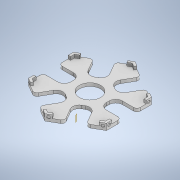
# Autodesk Inventor part: hexlight-bottom-led-module
Saved by Autodesk Inventor 2020 (Build 240168000, 168)
## iProperties
Created: 2019-10-02
Part Number: hexlight-bottom-led-module
Material: Generic
Document SubType Name: Modeling
Designer: Adam
Density: 1 g/cm^3
Appearance: Default
Author: Adam
Autodesk Inventor part; units mm, degrees
ref_plane "YZ Plane" through (0, 0, 0) normal (1, 0, 0) x (0, 1, 0)
ref_plane "XZ Plane" through (0, 0, 0) normal (0, 1, 0) x (-1, 0, 0)
ref_plane "XY Plane" through (0, 0, 0) normal (0, 0, 1) x (1, 0, 0)
sketch "Sketch1" plane through (0, 0, 0) normal (0, 1, 0) x (-1, 0, 0)
  line L0 (73.6122, 42.5) -> (73.6122, -42.5)
  line L1 (73.6122, -42.5) -> (0, -85)
  line L2 (0, -85) -> (-73.6122, -42.5)
  line L3 (-73.6122, -42.5) -> (-73.6122, 42.5)
  line L4 (-73.6122, 42.5) -> (0, 85)
  line L5 (0, 85) -> (73.6122, 42.5)
  point P0 (0, 0)
  point P1 (0, 0)
  dimension "d1" = 0
  dimension "d2" = 85
  constraints: 12 end point, 1 coincident, 13 other
  measures "d1" horizontal distance of point (0, 0) L4.end
  measures "d2" distance of L0.start L0.end
extrude "Extrusion1" add sketch "Sketch1" along normal blind 12
sketch "Sketch2" plane through (0, 12, 0) normal (0, 1, 0) x (1, 0, 0)
  line L0 (-69.282, -40) -> (-69.282, 40)
  line L1 (-69.282, 40) -> (0, 80)
  line L2 (0, 80) -> (69.282, 40)
  line L3 (69.282, 40) -> (69.282, -40)
  line L4 (69.282, -40) -> (0, -80)
  line L5 (0, -80) -> (-69.282, -40)
  point P0 (0, 0)
  point P1 (0, 0)
  dimension "d5" = 0
  dimension "d6" = 80
  constraints: 12 end point, 1 coincident, 13 other
  measures "d5" horizontal distance of point (0, 0) L4.end
  measures "d6" distance of L0.start L0.end
extrude "Extrusion2" cut sketch "Sketch2" against normal blind 6
sketch "Sketch6" plane through (73.6122, 0, 42.5) normal (0.5, 0, 0.8660254) x (0.8660254, 0, -0.5)
  line L0 (-75, 12) -> (-10, 12)
  line L1 (-10, 12) -> (-10, 6)
  line L2 (-10, 6) -> (-75, 6)
  line L3 (-75, 6) -> (-75, 12)
  line L4 (-85, 0) -> (0, 0) projected
  line L5 (-85, 12) -> (0, 12) projected
  line L6 (0, 0) -> (0, 12) projected
  line L7 (-85, 0) -> (-85, 12) projected
  line L8 (-82.5, 6) -> (-2.5, 6) projected
  point P0 (-42.5, 0)
  dimension "d34" = 0
  dimension "d35" = 10
  dimension "d36" = 10
  dimension "d37" = 0
  constraints: 8 end point, 2 parallel, 1 horizontal, 1 perpendicular
  measures "d34" distance between parallel lines of L5 L0
  measures "d35" distance between parallel lines of L6 L1
  measures "d36" distance between parallel lines of L7 L3
  measures "d37" distance between parallel lines of L8 L2
extrude "Extrusion4" cut sketch "Sketch6" against normal blind 11 contours L0 L1 L2 L3
pattern_circular "Circular Pattern2" count 6 over 360 about axis through (0, -10, 0) along (0, 1, 0) of "Extrusion4"
sketch "Sketch7" plane through (0, 0, 85) normal (0.5, 0, 0.8660254) x (0.8660254, 0, -0.5)
  line L0 (0, 0) -> (0, 12) projected
  line L1 (0, 12) -> (10, 12) projected
  point P0 (42.5, 0)
  point P1 (5, 7)
  dimension "d43" = 5
  dimension "d44" = 5
  measures "d43" distance from line of L0 point (5, 7)
  measures "d44" distance from line of L1 point (5, 7)
hole "Hole2" at (4.3301, 7, 82.5) direction (-0.5, 0, -0.8660254) diameter 5.5 depth 1.5
ref_plane "Work Plane1" through (36.8061, 6, 63.75) normal (0.8660254, 0, -0.5) x (-0.5, 0, -0.8660254)
mirror "Mirror1" about plane through (36.8061, 6, 63.75) normal (0.8660254, 0, -0.5) of "Hole2"
pattern_circular "Circular Pattern3" count 6 over 360 about axis through (0, -10, 0) along (0, 1, 0) of "Hole2", "Mirror1"
sketch "Sketch9" plane through (0, 0, 0) normal (0, -1, 0) x (1, 0, 0)
  line L0 (73.6122, 15) -> (46.1122, 15)
  line L1 (33.6122, 2.5) -> (33.6122, -2.5)
  line L2 (46.1122, -15) -> (73.6122, -15)
  line L3 (73.6122, -15) -> (73.6122, 15)
  line L4 (73.6122, 42.5) -> (73.6122, -42.5) projected
  arc A0 (33.6122, -2.5) -> (46.1122, -15) centre (46.1122, -2.5) ccw
  arc A1 (46.1122, 15) -> (33.6122, 2.5) centre (46.1122, 2.5) ccw
  point P0 (0, 0)
  dimension "d64" = 0
  dimension "d65" = 15
  dimension "d67" = 15
  dimension "d68" = 40
  dimension "d71" = 25
  dimension "d72" = 25
  constraints: 8 end point, 4 point on circle, 4 tangent, 2 centre point, 2 parallel, 1 horizontal, 1 perpendicular
  measures "d64" distance between parallel lines of L4 L3
  measures "d65" distance from line of point (0, 0) L0
  measures "d67" distance from line of point (0, 0) L2
  measures "d68" distance between parallel lines of L1 L3
  measures "d71" diameter of A0
  measures "d72" diameter of A1
extrude "Extrusion6" cut sketch "Sketch9" against normal blind 6
sketch "Sketch10" plane through (0, 0, 0) normal (0, -1, 0) x (1, 0, 0)
  line L0 (-17.6122, 27) -> (17.3878, 27) construction
  line L1 (17.3878, 27) -> (17.3878, 20.1168) construction
  line L2 (17.3878, 20.1168) -> (-17.6122, 20.1168) construction
  line L3 (-17.6122, 20.1168) -> (-17.6122, 27) construction
  line L4 (-73.6122, -42.5) -> (-73.6122, 42.5) projected
  line L5 (-73.6122, 42.5) -> (0, 85) projected
  line L6 (0, -85) -> (-73.6122, -42.5) projected
  line L7 (-15.0903, 23.8977) -> (-15.4954, 23.8977)
  line L8 (-15.4954, 23.8977) -> (-15.4954, 25.3895)
  line L9 (-15.4954, 25.3895) -> (-16.8983, 25.3895)
  line L10 (-16.8983, 25.3895) -> (-16.8983, 23.8977)
  line L11 (-16.8983, 23.8977) -> (-17.3034, 23.8977)
  line L12 (-17.3034, 23.8977) -> (-17.3034, 26.9457)
  line L13 (-17.3034, 26.9457) -> (-16.8983, 26.9457)
  line L14 (-16.8983, 26.9457) -> (-16.8983, 25.7502)
  line L15 (-16.8983, 25.7502) -> (-15.4954, 25.7502)
  line L16 (-15.4954, 25.7502) -> (-15.4954, 26.9457)
  line L17 (-15.4954, 26.9457) -> (-15.0903, 26.9457)
  line L18 (-15.0903, 26.9457) -> (-15.0903, 23.8977)
  line L19 (-14.4728, 23.8977) -> (-14.4728, 26.9457)
  line L20 (-14.4728, 26.9457) -> (-12.5659, 26.9457)
  line L21 (-12.5659, 26.9457) -> (-12.5659, 26.585)
  line L22 (-12.5659, 26.585) -> (-14.0677, 26.585)
  line L23 (-14.0677, 26.585) -> (-14.0677, 25.7502)
  line L24 (-14.0677, 25.7502) -> (-12.6672, 25.7502)
  line L25 (-12.6672, 25.7502) -> (-12.6672, 25.3895)
  line L26 (-12.6672, 25.3895) -> (-14.0677, 25.3895)
  line L27 (-14.0677, 25.3895) -> (-14.0677, 24.2583)
  line L28 (-14.0677, 24.2583) -> (-12.5659, 24.2583)
  line L29 (-12.5659, 24.2583) -> (-12.5659, 23.8977)
  line L30 (-12.5659, 23.8977) -> (-14.4728, 23.8977)
  line L31 (-10.0144, 23.8977) -> (-10.4788, 23.8977)
  line L32 (-10.4788, 23.8977) -> (-11.2198, 25.1129)
  line L33 (-11.2198, 25.1129) -> (-11.9756, 23.8977)
  line L34 (-11.9756, 23.8977) -> (-12.4128, 23.8977)
  line L35 (-12.4128, 23.8977) -> (-11.4421, 25.4241)
  line L36 (-11.4421, 25.4241) -> (-12.3831, 26.9457)
  line L37 (-12.3831, 26.9457) -> (-11.9188, 26.9457)
  line L38 (-11.9188, 26.9457) -> (-11.1926, 25.7526)
  line L39 (-11.1926, 25.7526) -> (-10.4516, 26.9457)
  line L40 (-10.4516, 26.9457) -> (-10.0144, 26.9457)
  line L41 (-10.0144, 26.9457) -> (-10.9678, 25.4439)
  line L42 (-10.9678, 25.4439) -> (-10.0144, 23.8977)
  line L43 (-7.9223, 23.8977) -> (-9.6883, 23.8977)
  line L44 (-9.6883, 23.8977) -> (-9.6883, 26.9457)
  line L45 (-9.6883, 26.9457) -> (-9.2833, 26.9457)
  line L46 (-9.2833, 26.9457) -> (-9.2833, 24.2583)
  line L47 (-9.2833, 24.2583) -> (-7.9223, 24.2583)
  line L48 (-7.9223, 24.2583) -> (-7.9223, 23.8977)
  line L49 (-6.5415, 23.8977) -> (-7.7222, 23.8977)
  line L50 (-7.7222, 23.8977) -> (-7.7222, 24.2089)
  line L51 (-7.7222, 24.2089) -> (-7.3344, 24.2089)
  line L52 (-7.3344, 24.2089) -> (-7.3344, 26.6344)
  line L53 (-7.3344, 26.6344) -> (-7.7222, 26.6344)
  line L54 (-7.7222, 26.6344) -> (-7.7222, 26.9457)
  line L55 (-7.7222, 26.9457) -> (-6.5415, 26.9457)
  line L56 (-6.5415, 26.9457) -> (-6.5415, 26.6344)
  line L57 (-6.5415, 26.6344) -> (-6.9293, 26.6344)
  line L58 (-6.9293, 26.6344) -> (-6.9293, 24.2089)
  line L59 (-6.9293, 24.2089) -> (-6.5415, 24.2089)
  line L60 (-6.5415, 24.2089) -> (-6.5415, 23.8977)
  spline S0 degree 2 poles (-4.7631, 23.8384) (-5.0867, 23.8384) (-5.6227, 24.036) (-5.8154, 24.2361) knots 0 0 0 1 2 2 2
  spline S1 degree 2 poles (-5.8154, 24.2361) (-6.008, 24.4386) (-6.213, 25.0363) (-6.213, 25.4241) knots 0 0 0 1 2 2 2
  spline S2 degree 2 poles (-6.213, 25.4241) (-6.213, 25.7922) (-6.0056, 26.3751) (-5.8129, 26.5826) knots 0 0 0 1 2 2 2
  spline S3 degree 2 poles (-5.8129, 26.5826) (-5.6276, 26.7826) (-5.0842, 27) (-4.7607, 27) knots 0 0 0 1 2 2 2
  spline S4 degree 2 poles (-4.7607, 27) (-4.6051, 27) (-4.3235, 26.9555) (-4.195, 26.916) knots 0 0 0 1 2 2 2
  spline S5 degree 2 poles (-4.195, 26.916) (-4.0913, 26.8864) (-3.8393, 26.7777) (-3.7628, 26.7382) knots 0 0 0 1 2 2 2
  line L61 (-3.7628, 26.7382) -> (-3.7628, 26.2491)
  line L62 (-3.7628, 26.2491) -> (-3.7974, 26.2491)
  spline S6 degree 2 poles (-3.7974, 26.2491) (-3.8739, 26.3158) (-4.0345, 26.4368) (-4.1827, 26.506) knots 0 0 0 1 2 2 2
  spline S7 degree 2 poles (-4.1827, 26.506) (-4.3062, 26.5677) (-4.6248, 26.6493) (-4.8076, 26.6493) knots 0 0 0 1 2 2 2
  spline S8 degree 2 poles (-4.8076, 26.6493) (-5.2473, 26.6493) (-5.7907, 25.9873) (-5.7907, 25.4365) knots 0 0 0 1 2 2 2
  spline S9 degree 2 poles (-5.7907, 25.4365) (-5.7907, 25.1302) (-5.6474, 24.6708) (-5.5115, 24.5127) knots 0 0 0 1 2 2 2
  spline S10 degree 2 poles (-5.5115, 24.5127) (-5.3806, 24.3546) (-5.0101, 24.1891) (-4.778, 24.1891) knots 0 0 0 1 2 2 2
  spline S11 degree 2 poles (-4.778, 24.1891) (-4.6075, 24.1891) (-4.2667, 24.2385) (-4.1506, 24.2879) knots 0 0 0 1 2 2 2
  line L63 (-4.1506, 24.2879) -> (-4.1506, 25.0759)
  line L64 (-4.1506, 25.0759) -> (-4.857, 25.0759)
  line L65 (-4.857, 25.0759) -> (-4.857, 25.4315)
  line L66 (-4.857, 25.4315) -> (-3.7504, 25.4315)
  line L67 (-3.7504, 25.4315) -> (-3.7504, 24.1002)
  spline S12 degree 2 poles (-3.7504, 24.1002) (-3.827, 24.0656) (-4.0888, 23.9594) (-4.2, 23.9273) knots 0 0 0 1 2 2 2
  spline S13 degree 2 poles (-4.2, 23.9273) (-4.3506, 23.8828) (-4.5927, 23.8384) (-4.7631, 23.8384) knots 0 0 0 1 2 2 2
  line L68 (-1.0285, 23.8977) -> (-1.4336, 23.8977)
  line L69 (-1.4336, 23.8977) -> (-1.4336, 25.3895)
  line L70 (-1.4336, 25.3895) -> (-2.8365, 25.3895)
  line L71 (-2.8365, 25.3895) -> (-2.8365, 23.8977)
  line L72 (-2.8365, 23.8977) -> (-3.2416, 23.8977)
  line L73 (-3.2416, 23.8977) -> (-3.2416, 26.9457)
  line L74 (-3.2416, 26.9457) -> (-2.8365, 26.9457)
  line L75 (-2.8365, 26.9457) -> (-2.8365, 25.7502)
  line L76 (-2.8365, 25.7502) -> (-1.4336, 25.7502)
  line L77 (-1.4336, 25.7502) -> (-1.4336, 26.9457)
  line L78 (-1.4336, 26.9457) -> (-1.0285, 26.9457)
  line L79 (-1.0285, 26.9457) -> (-1.0285, 23.8977)
  line L80 (0.3004, 23.8977) -> (0.3004, 26.585)
  line L81 (0.3004, 26.585) -> (-0.7222, 26.585)
  line L82 (-0.7222, 26.585) -> (-0.7222, 26.9457)
  line L83 (-0.7222, 26.9457) -> (1.7281, 26.9457)
  line L84 (1.7281, 26.9457) -> (1.7281, 26.585)
  line L85 (1.7281, 26.585) -> (0.7055, 26.585)
  line L86 (0.7055, 26.585) -> (0.7055, 23.8977)
  line L87 (0.7055, 23.8977) -> (0.3004, 23.8977)
  line L88 (5.9592, 23.8977) -> (5.5541, 23.8977)
  line L89 (5.5541, 23.8977) -> (5.5541, 26.5233)
  line L90 (5.5541, 26.5233) -> (4.7588, 24.7375)
  line L91 (4.7588, 24.7375) -> (4.5118, 24.7375)
  line L92 (4.5118, 24.7375) -> (3.7238, 26.5233)
  line L93 (3.7238, 26.5233) -> (3.7238, 23.8977)
  line L94 (3.7238, 23.8977) -> (3.3459, 23.8977)
  line L95 (3.3459, 23.8977) -> (3.3459, 26.9457)
  line L96 (3.3459, 26.9457) -> (3.8992, 26.9457)
  line L97 (3.8992, 26.9457) -> (4.66, 25.2488)
  line L98 (4.66, 25.2488) -> (5.396, 26.9457)
  line L99 (5.396, 26.9457) -> (5.9592, 26.9457)
  line L100 (5.9592, 26.9457) -> (5.9592, 23.8977)
  line L101 (6.2482, 23.8977) -> (7.2757, 26.9457)
  line L102 (7.2757, 26.9457) -> (7.7747, 26.9457)
  line L103 (7.7747, 26.9457) -> (8.8022, 23.8977)
  line L104 (8.8022, 23.8977) -> (8.3749, 23.8977)
  line L105 (8.3749, 23.8977) -> (8.0982, 24.7498)
  line L106 (8.0982, 24.7498) -> (6.9349, 24.7498)
  line L107 (6.9349, 24.7498) -> (6.6582, 23.8977)
  line L108 (6.6582, 23.8977) -> (6.2482, 23.8977)
  line L109 (7.9871, 25.0956) -> (7.5153, 26.5307)
  line L110 (7.5153, 26.5307) -> (7.046, 25.0956)
  line L111 (7.046, 25.0956) -> (7.9871, 25.0956)
  line L112 (11.4501, 23.8977) -> (10.9239, 23.8977)
  line L113 (10.9239, 23.8977) -> (9.9606, 25.1104)
  line L114 (9.9606, 25.1104) -> (9.4963, 25.1104)
  line L115 (9.4963, 25.1104) -> (9.4963, 23.8977)
  line L116 (9.4963, 23.8977) -> (9.0912, 23.8977)
  line L117 (9.0912, 23.8977) -> (9.0912, 26.9457)
  line L118 (9.0912, 26.9457) -> (9.8767, 26.9457)
  spline S14 degree 2 poles (9.8767, 26.9457) (10.1385, 26.9457) (10.4917, 26.8888) (10.6522, 26.7851) knots 0 0 0 1 2 2 2
  spline S15 degree 2 poles (10.6522, 26.7851) (10.8128, 26.6814) (10.998, 26.3578) (10.998, 26.1182) knots 0 0 0 1 2 2 2
  spline S16 degree 2 poles (10.998, 26.1182) (10.998, 25.7848) (10.6572, 25.3327) (10.3657, 25.2241) knots 0 0 0 1 2 2 2
  line L119 (10.3657, 25.2241) -> (11.4501, 23.8977)
  spline S17 degree 2 poles (10.5757, 26.0861) (10.5757, 26.2195) (10.4818, 26.4245) (10.383, 26.4912) knots 0 0 0 1 2 2 2
  spline S18 degree 2 poles (10.383, 26.4912) (10.2966, 26.548) (10.0668, 26.5949) (9.8989, 26.5949) knots 0 0 0 1 2 2 2
  line L120 (9.8989, 26.5949) -> (9.4963, 26.5949)
  line L121 (9.4963, 26.5949) -> (9.4963, 25.4488)
  line L122 (9.4963, 25.4488) -> (9.852, 25.4488)
  spline S19 degree 2 poles (9.852, 25.4488) (10.0273, 25.4488) (10.3064, 25.5106) (10.4028, 25.6069) knots 0 0 0 1 2 2 2
  spline S20 degree 2 poles (10.4028, 25.6069) (10.4917, 25.6909) (10.5757, 25.928) (10.5757, 26.0861) knots 0 0 0 1 2 2 2
  line L123 (13.9151, 23.8977) -> (13.389, 23.8977)
  line L124 (13.389, 23.8977) -> (12.275, 25.3154)
  line L125 (12.275, 25.3154) -> (12.0972, 25.1154)
  line L126 (12.0972, 25.1154) -> (12.0972, 23.8977)
  line L127 (12.0972, 23.8977) -> (11.6921, 23.8977)
  line L128 (11.6921, 23.8977) -> (11.6921, 26.9457)
  line L129 (11.6921, 26.9457) -> (12.0972, 26.9457)
  line L130 (12.0972, 26.9457) -> (12.0972, 25.5452)
  line L131 (12.0972, 25.5452) -> (13.347, 26.9457)
  line L132 (13.347, 26.9457) -> (13.841, 26.9457)
  line L133 (13.841, 26.9457) -> (12.5788, 25.5847)
  line L134 (12.5788, 25.5847) -> (13.9151, 23.8977)
  line L135 (15.2193, 23.8977) -> (14.0386, 23.8977)
  line L136 (14.0386, 23.8977) -> (14.0386, 24.2089)
  line L137 (14.0386, 24.2089) -> (14.4264, 24.2089)
  line L138 (14.4264, 24.2089) -> (14.4264, 26.6344)
  line L139 (14.4264, 26.6344) -> (14.0386, 26.6344)
  line L140 (14.0386, 26.6344) -> (14.0386, 26.9457)
  line L141 (14.0386, 26.9457) -> (15.2193, 26.9457)
  line L142 (15.2193, 26.9457) -> (15.2193, 26.6344)
  line L143 (15.2193, 26.6344) -> (14.8315, 26.6344)
  line L144 (14.8315, 26.6344) -> (14.8315, 24.2089)
  line L145 (14.8315, 24.2089) -> (15.2193, 24.2089)
  line L146 (15.2193, 24.2089) -> (15.2193, 23.8977)
  line L147 (16.7828, 23.8977) -> (15.6021, 23.8977)
  line L148 (15.6021, 23.8977) -> (15.6021, 24.2089)
  line L149 (15.6021, 24.2089) -> (15.9899, 24.2089)
  line L150 (15.9899, 24.2089) -> (15.9899, 26.6344)
  line L151 (15.9899, 26.6344) -> (15.6021, 26.6344)
  line L152 (15.6021, 26.6344) -> (15.6021, 26.9457)
  line L153 (15.6021, 26.9457) -> (16.7828, 26.9457)
  line L154 (16.7828, 26.9457) -> (16.7828, 26.6344)
  line L155 (16.7828, 26.6344) -> (16.395, 26.6344)
  line L156 (16.395, 26.6344) -> (16.395, 24.2089)
  line L157 (16.395, 24.2089) -> (16.7828, 24.2089)
  line L158 (16.7828, 24.2089) -> (16.7828, 23.8977)
  point P0 (0, 0)
  point P1 (-73.6122, 15)
  point P2 (-23.8157, 71.25)
  point P3 (-23.8157, -71.25)
  dimension "d76" = 56
  dimension "d77" = 35
  dimension "d78" = 58
  constraints: 2 other
  measures "d76" distance between parallel lines of L4 L3
  measures "d77" distance from line of L0.end L3
  measures "d78" distance from line of L5.end L0
emboss "Emboss1" sketch "Sketch10" operation cut depth 0.2 direction (0, 1, 0)
sketch "Sketch11" plane through (0, 0, 0) normal (0, -1, 0) x (1, 0, 0)
  circle A0 centre (0, 0) radius 20
  dimension "d81" = 40
  constraints: 1 centre point, 1 coincident
  measures "d81" diameter of A0
extrude "Extrusion7" cut sketch "Sketch11" against normal blind 6
pattern_circular "Circular Pattern5" count 6 over 360 about axis through (0, -10, 0) along (0, 1, 0) of "Extrusion6"
fillet "Fillet6" radius 6 12 edges at (73.6122, 3, -15) (73.6122, 3, 15) (49.7965, 3, 56.25) (23.8157, 3, 71.25) (-23.8157, 3, 71.25) (-49.7965, 3, 56.25) (-73.6122, 3, 15) (-73.6122, 3, -15) (-49.7965, 3, -56.25) (-23.8157, 3, -71.25) (23.8157, 3, -71.25) (49.7965, 3, -56.25)
equation "\"d36\" = d35"
equation "\"d67\" = d65"
body "Solid1"
